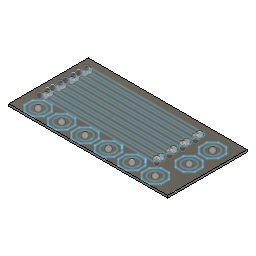
Zaagblad_A (Autodesk Fusion 360 archive; units mm, degrees)
design "Zaagblad_A_new" references "autodesk generic router xyz"
Autodesk Fusion 360 part; units mm, degrees
sketch "Board_1" plane through (0, 0, 0) normal (0, 0, 1) x (1, 0, 0)
  line L0 (0, 0) -> (1220, 0)
  line L1 (1220, 0) -> (1220, -610)
  line L2 (1220, -610) -> (0, -610)
  line L3 (0, -610) -> (0, 0)
  dimension "d1" = 1220
  dimension "d2" = 610
  constraint horizontal L0
  constraint vertical L1
  constraint horizontal L2
  constraint vertical L3
  constraint coincident L0.start L3.end
  measures "d1" distance of L0.start L0.end
  measures "d2" distance of L0.start L2.end
sketch "Board_1_piece_1" plane through (0, 0, 0) normal (0, 0, 1) x (1, 0, 0)
  line L0 (70, -120) -> (920, -120)
  line L1 (945, -95) -> (945, -90)
  line L2 (45, -90) -> (45, -95)
  arc A0 (45, -95) -> (70, -120) centre (70, -95) ccw
  arc A1 (920, -120) -> (945, -95) centre (920, -95) ccw
  line L3 (45, -90) -> (945, -90)
  line L4 (45, -70) -> (945, -70)
  line L5 (945, -70) -> (945, -65)
  arc A2 (945, -65) -> (920, -40) centre (920, -65) ccw
  line L6 (920, -40) -> (70, -40)
  arc A3 (70, -40) -> (45, -65) centre (70, -65) ccw
  line L7 (45, -65) -> (45, -70)
  arc A4 (70, -140) -> (45, -165) centre (70, -165) ccw
  line L8 (45, -190) -> (45, -195)
  arc A5 (45, -195) -> (70, -220) centre (70, -195) ccw
  line L9 (45, -190) -> (945, -190)
  line L10 (945, -170) -> (945, -165)
  line L11 (45, -165) -> (45, -170)
  line L12 (920, -140) -> (70, -140)
  line L13 (45, -170) -> (945, -170)
  arc A6 (945, -165) -> (920, -140) centre (920, -165) ccw
  line L14 (70, -220) -> (920, -220)
  arc A7 (920, -220) -> (945, -195) centre (920, -195) ccw
  line L15 (945, -195) -> (945, -190)
  line L16 (45, -270) -> (945, -270)
  line L17 (45, -290) -> (45, -295)
  arc A8 (920, -320) -> (945, -295) centre (920, -295) ccw
  arc A9 (70, -240) -> (45, -265) centre (70, -265) ccw
  line L18 (945, -295) -> (945, -290)
  line L19 (45, -290) -> (945, -290)
  line L20 (45, -265) -> (45, -270)
  line L21 (920, -240) -> (70, -240)
  line L22 (945, -270) -> (945, -265)
  arc A10 (45, -295) -> (70, -320) centre (70, -295) ccw
  arc A11 (945, -265) -> (920, -240) centre (920, -265) ccw
  line L23 (70, -320) -> (920, -320)
  line L24 (45, -390) -> (945, -390)
  arc A12 (920, -420) -> (945, -395) centre (920, -395) ccw
  line L25 (70, -420) -> (920, -420)
  arc A13 (70, -340) -> (45, -365) centre (70, -365) ccw
  line L26 (45, -365) -> (45, -370)
  arc A14 (945, -365) -> (920, -340) centre (920, -365) ccw
  line L27 (920, -340) -> (70, -340)
  line L28 (45, -370) -> (945, -370)
  line L29 (45, -390) -> (45, -395)
  arc A15 (45, -395) -> (70, -420) centre (70, -395) ccw
  line L30 (945, -395) -> (945, -390)
  line L31 (945, -370) -> (945, -365)
  point P0 (45, -120)
  point P1 (945, -120)
  point P2 (45, -60)
  point P3 (45, -220)
  point P4 (945, -220)
  point P5 (45, -160)
  point P6 (45, -320)
  point P7 (945, -320)
  point P8 (45, -260)
  point P9 (45, -420)
  point P10 (945, -420)
  point P11 (45, -360)
  dimension "d5" = 900
  dimension "d6" = 60
  dimension "d17" = 25
  dimension "d24" = 25
  dimension "d189" = 25
  dimension "d190" = 25
  dimension "d191" = 900
  dimension "d192" = 60
  dimension "d193" = 25
  dimension "d194" = 25
  dimension "d195" = 25
  dimension "d196" = 25
  dimension "d197" = 900
  dimension "d198" = 60
  dimension "d199" = 25
  dimension "d200" = 25
  dimension "d201" = 25
  dimension "d202" = 25
  dimension "d203" = 900
  dimension "d204" = 60
  dimension "d205" = 25
  dimension "d206" = 25
  dimension "d207" = 25
  dimension "d208" = 25
  constraint horizontal L0
  constraint vertical L1
  constraint vertical L2
  constraint coincident P2 L2
  constraint coincident P0 L0
  constraint coincident P0 L2
  constraint tangent L0 A0
  constraint tangent L2 A0
  constraint coincident P1 L0
  constraint coincident P1 L1
  constraint tangent L0 A1
  constraint tangent L1 A1
  constraint vertical L5
  constraint horizontal L6
  constraint vertical L7
  constraint tangent L6 A3
  constraint tangent A3 L7
  constraint tangent L5 A2
  constraint tangent A2 L6
  constraint horizontal L14
  constraint vertical L15
  constraint vertical L8
  constraint coincident P5 L8
  constraint coincident P3 L14
  constraint coincident P3 L8
  constraint tangent A5 L14
  constraint tangent L8 A5
  constraint coincident P4 L14
  constraint coincident P4 L15
  constraint tangent L14 A7
  constraint tangent A7 L15
  constraint vertical L10
  constraint horizontal L12
  constraint vertical L11
  constraint tangent A4 L12
  constraint tangent A4 L11
  constraint tangent L10 A6
  constraint tangent L12 A6
  constraint horizontal L23
  constraint vertical L18
  constraint vertical L17
  constraint coincident P8 L17
  constraint coincident P6 L23
  constraint coincident P6 L17
  constraint tangent A10 L23
  constraint tangent L17 A10
  constraint coincident P7 L23
  constraint coincident P7 L18
  constraint tangent A8 L23
  constraint tangent A8 L18
  constraint vertical L22
  constraint horizontal L21
  constraint vertical L20
  constraint tangent A9 L21
  constraint tangent A9 L20
  constraint tangent L22 A11
  constraint tangent L21 A11
  constraint horizontal L25
  constraint vertical L30
  constraint vertical L29
  constraint coincident P11 L29
  constraint coincident P9 L25
  constraint coincident P9 L29
  constraint tangent L25 A15
  constraint tangent L29 A15
  constraint coincident P10 L25
  constraint coincident P10 L30
  constraint tangent A12 L25
  constraint tangent A12 L30
  constraint vertical L31
  constraint horizontal L27
  constraint vertical L26
  constraint tangent A13 L27
  constraint tangent A13 L26
  constraint tangent A14 L31
  constraint tangent A14 L27
  measures "d5" distance of P0 P1
  measures "d6" distance of P0 P2
  measures "d17" radius of A0
  measures "d24" radius of A1
  measures "d189" radius of A3
  measures "d190" radius of A2
  measures "d191" distance of P3 P4
  measures "d192" distance of P3 P5
  measures "d193" radius of A5
  measures "d194" radius of A7
  measures "d195" radius of A4
  measures "d196" radius of A6
  measures "d197" distance of P6 P7
  measures "d198" distance of P6 P8
  measures "d199" radius of A10
  measures "d200" radius of A8
  measures "d201" radius of A9
  measures "d202" radius of A11
  measures "d203" distance of P9 P10
  measures "d204" distance of P9 P11
  measures "d205" radius of A15
  measures "d206" radius of A12
  measures "d207" radius of A13
  measures "d208" radius of A14
sketch "Board_3" plane through (0, 0, 0) normal (0, 0, 1) x (1, 0, 0)
sketch "Board_3_piece_1" plane through (0, 0, 0) normal (0, 0, 1) x (1, 0, 0)
sketch "Board_3_piece_2" plane through (0, 0, 0) normal (0, 0, 1) x (1, 0, 0)
  line L0 (1044.3853, -226.0896) -> (1105.6147, -226.0896)
  line L1 (1105.6147, -226.0896) -> (1148.9104, -269.3853)
  line L2 (1044.3853, -226.0896) -> (1105.6147, -226.0896)
  line L3 (1148.9104, -330.6147) -> (1105.6147, -373.9104)
  line L4 (1001.0896, -269.3853) -> (1044.3853, -226.0896)
  line L5 (1105.6147, -373.9104) -> (1044.3853, -373.9104)
  line L6 (1001.0896, -269.3853) -> (1044.3853, -226.0896)
  line L7 (1044.3853, -373.9104) -> (1001.0896, -330.6147)
  line L8 (1148.9104, -269.3853) -> (1148.9104, -330.6147)
  line L9 (1001.0896, -330.6147) -> (1001.0896, -269.3853)
  line L10 (1105.6147, -373.9104) -> (1044.3853, -373.9104)
  line L11 (1148.9104, -269.3853) -> (1148.9104, -330.6147)
  line L12 (1044.3853, -373.9104) -> (1001.0896, -330.6147)
  line L13 (1001.0896, -330.6147) -> (1001.0896, -269.3853)
  line L14 (1105.6147, -226.0896) -> (1148.9104, -269.3853)
  line L15 (1148.9104, -330.6147) -> (1105.6147, -373.9104)
  line L16 (94.3853, -436.0896) -> (155.6147, -436.0896)
  line L17 (155.6147, -583.9104) -> (94.3853, -583.9104)
  line L18 (51.0896, -540.6147) -> (51.0896, -479.3853)
  line L19 (198.9104, -540.6147) -> (155.6147, -583.9104)
  line L20 (198.9104, -540.6147) -> (155.6147, -583.9104)
  line L21 (94.3853, -583.9104) -> (51.0896, -540.6147)
  line L22 (155.6147, -583.9104) -> (94.3853, -583.9104)
  line L23 (94.3853, -436.0896) -> (155.6147, -436.0896)
  line L24 (198.9104, -479.3853) -> (198.9104, -540.6147)
  line L25 (51.0896, -540.6147) -> (51.0896, -479.3853)
  line L26 (94.3853, -583.9104) -> (51.0896, -540.6147)
  line L27 (198.9104, -479.3853) -> (198.9104, -540.6147)
  line L28 (155.6147, -436.0896) -> (198.9104, -479.3853)
  line L29 (51.0896, -479.3853) -> (94.3853, -436.0896)
  line L30 (51.0896, -479.3853) -> (94.3853, -436.0896)
  line L31 (155.6147, -436.0896) -> (198.9104, -479.3853)
  line L32 (335.6147, -436.0896) -> (378.9104, -479.3853)
  line L33 (335.6147, -436.0896) -> (378.9104, -479.3853)
  line L34 (335.6147, -583.9104) -> (274.3853, -583.9104)
  line L35 (378.9104, -540.6147) -> (335.6147, -583.9104)
  line L36 (274.3853, -583.9104) -> (231.0896, -540.6147)
  line L37 (274.3853, -583.9104) -> (231.0896, -540.6147)
  line L38 (274.3853, -436.0896) -> (335.6147, -436.0896)
  line L39 (231.0896, -479.3853) -> (274.3853, -436.0896)
  line L40 (231.0896, -540.6147) -> (231.0896, -479.3853)
  line L41 (231.0896, -479.3853) -> (274.3853, -436.0896)
  line L42 (378.9104, -540.6147) -> (335.6147, -583.9104)
  line L43 (378.9104, -479.3853) -> (378.9104, -540.6147)
  line L44 (378.9104, -479.3853) -> (378.9104, -540.6147)
  line L45 (274.3853, -436.0896) -> (335.6147, -436.0896)
  line L46 (231.0896, -540.6147) -> (231.0896, -479.3853)
  line L47 (335.6147, -583.9104) -> (274.3853, -583.9104)
  line L48 (515.6147, -583.9104) -> (454.3853, -583.9104)
  line L49 (515.6147, -583.9104) -> (454.3853, -583.9104)
  line L50 (454.3853, -583.9104) -> (411.0896, -540.6147)
  line L51 (411.0896, -540.6147) -> (411.0896, -479.3853)
  line L52 (411.0896, -540.6147) -> (411.0896, -479.3853)
  line L53 (454.3853, -436.0896) -> (515.6147, -436.0896)
  line L54 (558.9104, -479.3853) -> (558.9104, -540.6147)
  line L55 (558.9104, -540.6147) -> (515.6147, -583.9104)
  line L56 (411.0896, -479.3853) -> (454.3853, -436.0896)
  line L57 (558.9104, -479.3853) -> (558.9104, -540.6147)
  line L58 (515.6147, -436.0896) -> (558.9104, -479.3853)
  line L59 (515.6147, -436.0896) -> (558.9104, -479.3853)
  line L60 (454.3853, -436.0896) -> (515.6147, -436.0896)
  line L61 (411.0896, -479.3853) -> (454.3853, -436.0896)
  line L62 (454.3853, -583.9104) -> (411.0896, -540.6147)
  line L63 (558.9104, -540.6147) -> (515.6147, -583.9104)
  line L64 (738.9104, -540.6147) -> (695.6147, -583.9104)
  line L65 (591.0896, -479.3853) -> (634.3853, -436.0896)
  line L66 (738.9104, -540.6147) -> (695.6147, -583.9104)
  line L67 (695.6147, -436.0896) -> (738.9104, -479.3853)
  line L68 (591.0896, -540.6147) -> (591.0896, -479.3853)
  line L69 (738.9104, -479.3853) -> (738.9104, -540.6147)
  line L70 (591.0896, -540.6147) -> (591.0896, -479.3853)
  line L71 (634.3853, -436.0896) -> (695.6147, -436.0896)
  line L72 (695.6147, -583.9104) -> (634.3853, -583.9104)
  line L73 (634.3853, -583.9104) -> (591.0896, -540.6147)
  line L74 (695.6147, -583.9104) -> (634.3853, -583.9104)
  line L75 (634.3853, -436.0896) -> (695.6147, -436.0896)
  line L76 (738.9104, -479.3853) -> (738.9104, -540.6147)
  line L77 (634.3853, -583.9104) -> (591.0896, -540.6147)
  line L78 (591.0896, -479.3853) -> (634.3853, -436.0896)
  line L79 (695.6147, -436.0896) -> (738.9104, -479.3853)
  line L80 (771.0896, -540.6147) -> (771.0896, -479.3853)
  line L81 (875.6147, -583.9104) -> (814.3853, -583.9104)
  line L82 (875.6147, -436.0896) -> (918.9104, -479.3853)
  line L83 (814.3853, -583.9104) -> (771.0896, -540.6147)
  line L84 (814.3853, -583.9104) -> (771.0896, -540.6147)
  line L85 (875.6147, -436.0896) -> (918.9104, -479.3853)
  line L86 (875.6147, -583.9104) -> (814.3853, -583.9104)
  line L87 (814.3853, -436.0896) -> (875.6147, -436.0896)
  line L88 (771.0896, -479.3853) -> (814.3853, -436.0896)
  line L89 (918.9104, -540.6147) -> (875.6147, -583.9104)
  line L90 (771.0896, -540.6147) -> (771.0896, -479.3853)
  line L91 (918.9104, -479.3853) -> (918.9104, -540.6147)
  line L92 (814.3853, -436.0896) -> (875.6147, -436.0896)
  line L93 (918.9104, -479.3853) -> (918.9104, -540.6147)
  line L94 (771.0896, -479.3853) -> (814.3853, -436.0896)
  line L95 (918.9104, -540.6147) -> (875.6147, -583.9104)
  line L96 (1055.6147, -436.0896) -> (1098.9104, -479.3853)
  line L97 (994.3853, -583.9104) -> (951.0896, -540.6147)
  line L98 (1055.6147, -583.9104) -> (994.3853, -583.9104)
  line L99 (1098.9104, -540.6147) -> (1055.6147, -583.9104)
  line L100 (1055.6147, -583.9104) -> (994.3853, -583.9104)
  line L101 (1098.9104, -479.3853) -> (1098.9104, -540.6147)
  line L102 (951.0896, -540.6147) -> (951.0896, -479.3853)
  line L103 (951.0896, -479.3853) -> (994.3853, -436.0896)
  line L104 (1055.6147, -436.0896) -> (1098.9104, -479.3853)
  line L105 (1098.9104, -479.3853) -> (1098.9104, -540.6147)
  line L106 (951.0896, -540.6147) -> (951.0896, -479.3853)
  line L107 (994.3853, -436.0896) -> (1055.6147, -436.0896)
  line L108 (994.3853, -583.9104) -> (951.0896, -540.6147)
  line L109 (994.3853, -436.0896) -> (1055.6147, -436.0896)
  line L110 (1098.9104, -540.6147) -> (1055.6147, -583.9104)
  line L111 (951.0896, -479.3853) -> (994.3853, -436.0896)
  line L112 (1044.3853, -193.9104) -> (1001.0896, -150.6147)
  line L113 (1044.3853, -193.9104) -> (1001.0896, -150.6147)
  line L114 (1105.6147, -193.9104) -> (1044.3853, -193.9104)
  line L115 (1105.6147, -46.0896) -> (1148.9104, -89.3853)
  line L116 (1001.0896, -150.6147) -> (1001.0896, -89.3853)
  line L117 (1105.6147, -46.0896) -> (1148.9104, -89.3853)
  line L118 (1001.0896, -89.3853) -> (1044.3853, -46.0896)
  line L119 (1148.9104, -89.3853) -> (1148.9104, -150.6147)
  line L120 (1044.3853, -46.0896) -> (1105.6147, -46.0896)
  line L121 (1148.9104, -89.3853) -> (1148.9104, -150.6147)
  line L122 (1044.3853, -46.0896) -> (1105.6147, -46.0896)
  line L123 (1001.0896, -150.6147) -> (1001.0896, -89.3853)
  line L124 (1148.9104, -150.6147) -> (1105.6147, -193.9104)
  line L125 (1105.6147, -193.9104) -> (1044.3853, -193.9104)
  line L126 (1001.0896, -89.3853) -> (1044.3853, -46.0896)
  line L127 (1148.9104, -150.6147) -> (1105.6147, -193.9104)
  circle A0 centre (1075, -120) radius 48.25
  circle A1 centre (1075, -300) radius 48.25
  circle A2 centre (1025, -510) radius 48.25
  circle A3 centre (845, -510) radius 48.25
  circle A4 centre (665, -510) radius 48.25
  circle A5 centre (485, -510) radius 48.25
  circle A6 centre (305, -510) radius 48.25
  circle A7 centre (125, -510) radius 48.25
  dimension "d219" = 96.5
  dimension "d220" = 96.5
  dimension "d221" = 96.5
  dimension "d222" = 96.5
  dimension "d223" = 96.5
  dimension "d224" = 96.5
  dimension "d225" = 96.5
  dimension "d226" = 96.5
  measures "d219" diameter of A0
  measures "d220" diameter of A1
  measures "d221" diameter of A2
  measures "d222" diameter of A3
  measures "d223" diameter of A4
  measures "d224" diameter of A5
  measures "d225" diameter of A6
  measures "d226" diameter of A7
extrude "Extrude1" add sketch "Board_1" along normal blind 18
